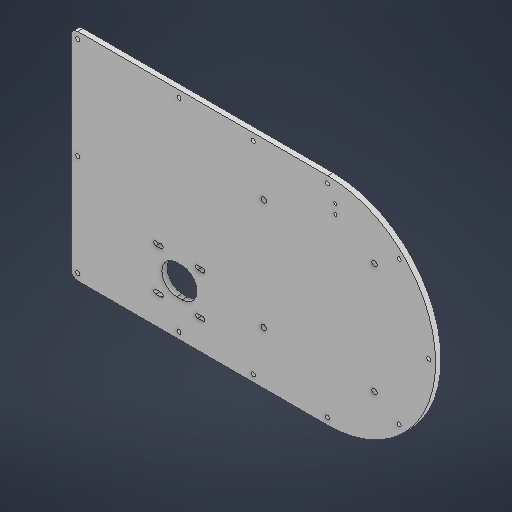
# Autodesk Inventor part: testbaseup
Saved by Autodesk Inventor 2025.2 (Build 292293000, 293)
## iProperties
Created: 2025-06-16
Part Number: testbaseup
Material: Generic
Document SubType Name: Modeling
Designer: Tiago
Density: 1 g/cm^3
Appearance: Default
Author: Tiago
Autodesk Inventor part; units mm, degrees
ref_plane "YZ Plane" through (0, 0, 0) normal (1, 0, 0) x (0, 1, 0)
ref_plane "XZ Plane" through (0, 0, 0) normal (0, 1, 0) x (-1, 0, 0)
ref_plane "XY Plane" through (0, 0, 0) normal (0, 0, 1) x (1, 0, 0)
sketch "Sketch1" plane through (0, 0, 0) normal (0, 0, 1) x (1, 0, 0)
  line L0 (-178.79, -80) -> (6.21, -80)
  line L1 (6.21, 80) -> (-178.79, 80)
  line L2 (-183.79, 75) -> (-183.79, -75)
  circle A0 centre (41, 41) radius 2
  circle A1 centre (41, -41) radius 2
  circle A2 centre (-41, -41) radius 2
  circle A3 centre (-41, 41) radius 2
  line L3 (86.21, 0) -> (86.21, 0)
  arc A4 (6.21, -80) -> (86.21, 0) centre (6.21, 0) ccw
  arc A5 (86.21, 0) -> (6.21, 80) centre (6.21, 0) ccw
  circle A6 centre (81.21, 0) radius 1.5
  circle A7 centre (59.243, -53.033) radius 1.5
  circle A8 centre (6.21, -75) radius 1.5
  circle A9 centre (-48.79, -75) radius 1.5
  circle A10 centre (-103.79, -75) radius 1.5
  circle A11 centre (-178.79, -75) radius 1.5
  circle A12 centre (-178.79, 0) radius 1.5
  circle A13 centre (-178.79, 75) radius 1.5
  circle A14 centre (-103.79, 75) radius 1.5
  circle A15 centre (-48.79, 75) radius 1.5
  circle A16 centre (6.21, 75) radius 1.5
  circle A17 centre (59.243, 53.033) radius 1.5
  circle A18 centre (12, 65) radius 1.1
  circle A19 centre (12, 58) radius 1.1
  arc A20 (-117.0042, -28.5) -> (-117.0042, -25.5) centre (-117.0042, -27) ccw
  line L4 (-117.0042, -28.5) -> (-121.0042, -28.5)
  line L5 (-117.0042, -25.5) -> (-121.0042, -25.5)
  arc A21 (-121.0042, -25.5) -> (-121.0042, -28.5) centre (-121.0042, -27) ccw
  arc A22 (-121.0042, -56.5) -> (-121.0042, -59.5) centre (-121.0042, -58) ccw
  line L6 (-117.0042, -59.5) -> (-121.0042, -59.5)
  line L7 (-117.0042, -56.5) -> (-121.0042, -56.5)
  arc A23 (-117.0042, -59.5) -> (-117.0042, -56.5) centre (-117.0042, -58) ccw
  arc A24 (-105.5042, -31.5) -> (-105.5042, -53.5) centre (-105.5042, -42.5) ccw
  arc A25 (-101.5042, -53.5) -> (-101.5042, -31.5) centre (-101.5042, -42.5) ccw
  line L8 (-101.5042, -31.5) -> (-105.5042, -31.5)
  line L9 (-101.5042, -53.5) -> (-105.5042, -53.5)
  arc A26 (-86.0042, -28.5) -> (-86.0042, -25.5) centre (-86.0042, -27) ccw
  line L10 (-86.0042, -28.5) -> (-90.0042, -28.5)
  line L11 (-86.0042, -25.5) -> (-90.0042, -25.5)
  arc A27 (-90.0042, -25.5) -> (-90.0042, -28.5) centre (-90.0042, -27) ccw
  arc A28 (-86.0042, -59.5) -> (-86.0042, -56.5) centre (-86.0042, -58) ccw
  line L12 (-86.0042, -59.5) -> (-90.0042, -59.5)
  line L13 (-86.0042, -56.5) -> (-90.0042, -56.5)
  arc A29 (-90.0042, -56.5) -> (-90.0042, -59.5) centre (-90.0042, -58) ccw
  arc A30 (-183.79, -75) -> (-178.79, -80) centre (-178.79, -75) ccw
  arc A31 (-178.79, 80) -> (-183.79, 75) centre (-178.79, 75) ccw
  point P0 (0, 0)
  point P1 (-183.79, -80)
  point P2 (-183.79, 80)
  point P3 (0, 0)
  point P4 (86.21, 0)
  point P5 (-103.5042, -42.5)
  point P6 (-103.5042, -42.5)
  point P7 (86.21, 0)
  point P8 (-119.0042, -58)
  point P9 (-103.5042, -42.5)
  point P10 (-103.5042, -53.5)
  point P11 (-119.0042, -25.5)
  point P12 (-119.0042, -28.5)
  dimension "d5" = 4
  dimension "d10" = 80
  dimension "d12" = 3
  dimension "d15" = 3
  dimension "d17" = 3
  dimension "d21" = 3
  dimension "d22" = 3
  dimension "d23" = 3
  dimension "d24" = 3
  dimension "d39" = 3
  dimension "d40" = 1.5
  dimension "d41" = 22
  dimension "d42" = 11
  dimension "d44" = 80
  dimension "d45" = 6.21
  dimension "d46" = 183.79
  dimension "d51" = 3
  dimension "d56" = 5
  dimension "d57" = 5
  dimension "d58" = 5
  dimension "d59" = 5
  dimension "d60" = 3
  dimension "d61" = 3
  dimension "d62" = 5
  dimension "d63" = 80
  dimension "d64" = 5
  dimension "d65" = 3
  dimension "d66" = 4
  dimension "d67" = 135
  dimension "d68" = 41
  dimension "d91" = 3
  dimension "d92" = 1.5
  dimension "d96" = 3
  dimension "d97" = 1.5
  dimension "d99" = 41
  dimension "d100" = 82
  dimension "d101" = 4
  dimension "d102" = 4
  dimension "d103" = 82
  dimension "d104" = 7
  dimension "d105" = 3
  dimension "d106" = 6.21
  dimension "d107" = 58
  dimension "d108" = 12
  dimension "d109" = 2.2
  dimension "d110" = 2.2
  dimension "d113" = 37.5
  dimension "d114" = 80.2858
  dimension "d115" = 2
  dimension "d116" = 2
  dimension "d117" = 80.2858
  dimension "d118" = 37.5
  dimension "d119" = 11
  dimension "d120" = 4
  dimension "d124" = 4
  dimension "d125" = 3
  dimension "d126" = 15.5
  dimension "d127" = 15.5
  dimension "d128" = 1.5
  dimension "d129" = 13.5
  dimension "d130" = 2
  dimension "d131" = 2
  dimension "d132" = 1.5
  dimension "d133" = 1.5
  constraints: 32 centre point, 28 end point, 28 point on circle, 24 tangent, 12 horizontal alignment, 6 vertical alignment, 5 coincident, 4 midpoint, 4 point on line, 2 equal radius, 1 horizontal, 1 parallel, 1 perpendicular
  measures "d5" diameter of A0
  measures "d10" radius of A4
  measures "d12" diameter of A6
  measures "d15" diameter of A7
  measures "d17" diameter of A8
  measures "d21" diameter of A9
  measures "d22" diameter of A10
  measures "d23" diameter of A11
  measures "d24" diameter of A12
  measures "d39" diameter of A20
  measures "d40" radius of A21
  measures "d41" diameter of A24
  measures "d42" radius of A25
  measures "d44" distance from line of point (0, 0) L0
  measures "d45" distance of A4.centre point (0, 0)
  measures "d46" distance from line of point (0, 0) L2
  measures "d51" diameter of A17
  measures "d56" distance from line of L2 A11.centre
  measures "d57" distance from line of L0 A11.centre
  measures "d58" distance from line of L2 A13.centre
  measures "d59" distance from line of L1 A13.centre
  measures "d60" diameter of A13
  measures "d61" diameter of A14
  measures "d62" distance from line of L1 A14.centre
  measures "d63" distance from line of L2 A14.centre
  measures "d64" distance from line of L1 A15.centre
  measures "d65" diameter of A15
  measures "d66" diameter of A3
  measures "d67" distance from line of L2 A15.centre
  measures "d68" horizontal distance of point (0, 0) A3.centre
  measures "d91" diameter of A26
  measures "d92" radius of A27
  measures "d96" diameter of A28
  measures "d97" radius of A29
  measures "d99" horizontal distance of A3.centre point (0, 0)
  measures "d100" distance of A3.centre A2.centre
  measures "d101" diameter of A2
  measures "d102" diameter of A1
  measures "d103" distance of A3.centre A0.centre
  measures "d104" distance of A18.centre A19.centre
  measures "d105" diameter of A16
  measures "d106" horizontal distance of point (0, 0) A16.centre
  measures "d107" vertical distance of point (0, 0) A19.centre
  measures "d108" horizontal distance of point (0, 0) A19.centre
  measures "d109" diameter of A18
  measures "d110" diameter of A19
  measures "d113" distance from line of L0 point (-103.504, -42.5)
  measures "d114" distance from line of L2 point (-103.504, -42.5)
  measures "d115" distance of A25.centre point (-103.504, -42.5)
  measures "d116" distance of A24.centre point (-103.504, -42.5)
  measures "d117" distance from line of L2 point (-103.504, -42.5)
  measures "d118" distance from line of L0 point (-103.504, -42.5)
  measures "d119" distance of point (-103.504, -53.5) point (-103.504, -42.5)
  measures "d120" distance of L8.start L8.end
  measures "d124" distance of A21.centre A20.centre
  measures "d125" distance of point (-119.004, -25.5) point (-119.004, -28.5)
  measures "d126" vertical distance of point (-103.504, -42.5) A20.centre
  measures "d127" vertical distance of point (-103.504, -42.5) A21.centre
  measures "d128" radius of A20
  measures "d129" horizontal distance of point (-103.504, -42.5) A20.centre
  measures "d130" distance of A23.centre point (-119.004, -58)
  measures "d131" distance of point (-119.004, -58) A22.centre
  measures "d132" radius of A22
  measures "d133" radius of A23
extrude "Extrusion1" add sketch "Sketch1" along normal blind 4
equation "\"d15\" = d12"
equation "\"d17\" = d12"
equation "\"d21\" = d12"
equation "\"d22\" = d12"
equation "\"d23\" = d12"
equation "\"d24\" = d12"
equation "\"d39\" = d31"
equation "\"d40\" = 0.5 * d31"
equation "\"d41\" = d9"
equation "\"d42\" = 0.5 * d9"
equation "\"d91\" = d89"
equation "\"d92\" = 0.5 * d89"
equation "\"d96\" = d94"
equation "\"d97\" = 0.5 * d94"
equation "\"d31\" = 3"
equation "\"d9\" = 22"
equation "\"d89\" = 3"
equation "\"d94\" = 3"
body "Solid1"
